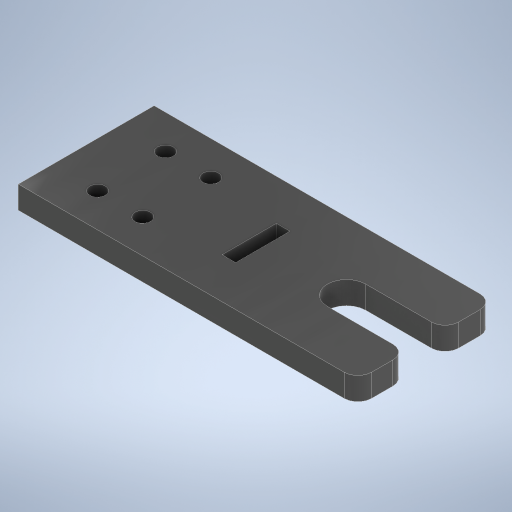
# Autodesk Inventor part: HCMUTE-CDT23-BAT_TRUC_CANG_TAI
Saved by Autodesk Inventor 2023 (Build 270158000, 158)
## iProperties
Created: 2023-11-19
Part Number: HCMUTE-CDT23-BAT_TRUC_CANG_TAI
Material: Stainless Steel
Document SubType Name: Sheet Metal
Designer: havie
Density: 8 g/cm^3
Sheet Metal Rule: Default_mm
Appearance: Dark Gray
Author: havie
Autodesk Inventor part; units mm, degrees
ref_plane "YZ Plane" through (0, 0, 0) normal (1, 0, 0) x (0, 1, 0)
ref_plane "XZ Plane" through (0, 0, 0) normal (0, 1, 0) x (-1, 0, 0)
ref_plane "XY Plane" through (0, 0, 0) normal (0, 0, 1) x (1, 0, 0)
sketch "Sketch1" plane through (0, 0, 0) normal (0, 1, 0) x (-1, 0, 0)
  line L0 (-75, 30) -> (75, 30)
  line L1 (75, 30) -> (75, -30)
  line L2 (75, -30) -> (-75, -30)
  line L3 (-75, -30) -> (-75, 30)
  line L4 (-75, 30) -> (75, -30) construction
  line L5 (75, 30) -> (-75, -30) construction
  line L6 (-80, 0) -> (-40, 0) construction
  line L7 (-80, -8.5) -> (-40, -8.5)
  line L8 (-40, 8.5) -> (-80, 8.5)
  arc A0 (-80, 8.5) -> (-80, -8.5) centre (-80, 0) ccw
  arc A1 (-40, -8.5) -> (-40, 8.5) centre (-40, 0) ccw
  circle A2 centre (55, 15) radius 3.5
  circle A3 centre (55, -15) radius 3.5
  circle A4 centre (35, 15) radius 3.5
  circle A5 centre (35, -15) radius 3.5
  point P0 (0, 0)
  point P1 (-60, 0)
  dimension "d0" = 60
  dimension "d1" = 150
  dimension "d2" = 60
  dimension "d3" = 40
  dimension "d4" = 17
  dimension "d5" = 7
  dimension "d6" = 15
  dimension "d7" = 30
  dimension "d8" = 20
  dimension "d9" = 20
  constraints: 20 end point, 6 centre point, 4 point on circle, 4 tangent, 3 equal radius, 3 horizontal alignment, 3 midpoint, 3 parallel, 2 horizontal, 2 vertical alignment, 1 perpendicular
  measures "d0" distance of L0.end L1.end
  measures "d1" distance of L1.end L2.end
  measures "d2" distance of point (0, 0) point (-60, 0)
  measures "d3" distance of L8.start L8.end
  measures "d4" distance between parallel lines of L7 L8
  measures "d5" diameter of A5
  measures "d6" distance from line of L0 A2.centre
  measures "d7" distance of A3.centre A2.centre
  measures "d8" distance from line of L1 A2.centre
  measures "d9" distance of A2.centre A4.centre
extrude "Plate1" add sketch "Sketch1" along normal mid plane 10 contours L0 L1 L2 L3 L7 A1 L8 | L8 A1 L7 L3
extrude "Cut1" cut sketch "Sketch1" against normal mid plane 10 contours L8 A1 L7 L3 | L3 L7 A0 L8
sketch "Sketch2" plane through (0, -5, 0) normal (0, -1, 0) x (1, 0, 0)
  line L0 (-3, 12) -> (3, 12)
  line L1 (3, 12) -> (3, -12)
  line L2 (3, -12) -> (-3, -12)
  line L3 (-3, -12) -> (-3, 12)
  line L4 (75, 30) -> (-75, 30) projected
  point P0 (0, 0)
  point P1 (0, 12)
  dimension "d13" = 24
  dimension "d14" = 18
  dimension "d15" = 6
  constraints: 8 end point, 2 parallel, 1 horizontal, 1 midpoint, 1 perpendicular, 1 vertical alignment
  measures "d13" distance of L0.end L1.end
  measures "d14" distance between parallel lines of L4 L0
  measures "d15" distance of L0.start L0.end
extrude "Cut2" cut sketch "Sketch2" against normal blind 10
fillet "Corner Round1" radius 6 4 edges at (75, 0, 30) (75, 0, 8.5) (75, 0, -8.5) (75, 0, -30)
equation "\"d11\" = Thickness"
equation "\"d16\" = Thickness"
equation "\"d10\" = Thickness"
equation "\"BendReliefDepth\" = 0.5 * Thickness"
equation "\"Thickness\" = 10"
body "Solid1"
